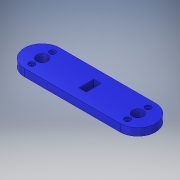
# Autodesk Inventor part: Middle_leg_a
Saved by Autodesk Inventor 2017 (Build 210142000, 142)
## iProperties
Created: 2016-06-08
Part Number: Middle_leg_a
Material: Generic
Document SubType Name: Modeling
Designer: alex-
Density: 1 g/cm^3
Appearance: Blue - Wall Paint - Glossy
Author: alex-
Autodesk Inventor part; units mm, degrees
ref_plane "YZ Plane" through (0, 0, 0) normal (1, 0, 0) x (0, 1, 0)
ref_plane "XZ Plane" through (0, 0, 0) normal (0, 1, 0) x (-1, 0, 0)
ref_plane "XY Plane" through (0, 0, 0) normal (0, 0, 1) x (1, 0, 0)
sketch "Sketch1" plane through (0, 0, 0) normal (0, 1, 0) x (-1, 0, 0)
  circle A0 centre (32.5, 0) radius 12
  circle A1 centre (-32.5, 0) radius 12
  line L0 (32.5, 12) -> (-32.5, 12)
  line L1 (32.5, -12) -> (-32.5, -12)
  circle A2 centre (32.5, 0) radius 3.75
  circle A3 centre (-32.5, 0) radius 3.75
  line L2 (62.3, 0) -> (-62.3, 0) projected
  circle A4 centre (32.5, -7) radius 1
  circle A5 centre (32.5, 7) radius 1
  circle A6 centre (-32.5, -7) radius 1
  circle A7 centre (-32.5, 7) radius 1
  line L3 (2.5, -5) -> (-2.5, -5)
  line L4 (-2.5, -5) -> (-2.5, 5)
  line L5 (-2.5, 5) -> (2.5, 5)
  line L6 (2.5, 5) -> (2.5, -5)
  point P0 (0, 0)
  point P1 (0, 12)
  point P2 (2.5, 0)
  point P3 (0, -5)
  dimension "d5" = 65
  dimension "d6" = 24
  dimension "d7" = 7.5
  dimension "d17" = 2
  dimension "d18" = 7
  dimension "d19" = 7
  dimension "d25" = 5
  dimension "d26" = 10
  constraints: 12 end point, 8 centre point, 6 vertical alignment, 5 equal radius, 5 horizontal alignment, 4 point on circle, 3 midpoint, 3 parallel, 2 coincident, 2 horizontal, 2 tangent, 1 perpendicular
  measures "d5" distance of A1.centre A0.centre
  measures "d6" diameter of A0
  measures "d7" diameter of A2
  measures "d17" diameter of A4
  measures "d18" distance of A0.centre A4.centre
  measures "d19" distance of A0.centre A5.centre
  measures "d25" distance of L3.start L3.end
  measures "d26" distance of L5.end L3.start
extrude "Extrusion7" add sketch "Sketch1" along normal blind 5 contours L2 A2 A0 | A0 L2 A2 | A0 L2 L6 L5 L4 A1 L0 | L1 A1 L2 L4 L3 L6 A0 | A1 L2 A3 | A1 L2 A3
sketch "Sketch4" plane through (0, 5, 0) normal (0, 1, 0) x (1, 0, 0)
  circle A0 centre (-32.5, -7) radius 2
  circle A1 centre (-32.5, 7) radius 2
  circle A2 centre (32.5, -7) radius 2
  circle A3 centre (32.5, 7) radius 2
  circle A4 centre (-32.5, -7) radius 1 projected
  circle A5 centre (-32.5, 7) radius 1 projected
  circle A6 centre (32.5, -7) radius 1 projected
  circle A7 centre (32.5, 7) radius 1 projected
  point P0 (0, 0)
  dimension "d29" = 4
  constraints: 4 centre point, 4 concentric, 3 equal radius
  measures "d29" diameter of A0
extrude "Extrusion8" cut sketch "Sketch4" against normal blind 1
equation "\"d6\" = sa_diameter"
equation "\"d25\" = b_mat_thickness"
equation "\"d27\" = b_mat_thickness"
equation "\"sa_diameter\" = 24"
equation "\"b_mat_thickness\" = 5"
body "Solid4"
